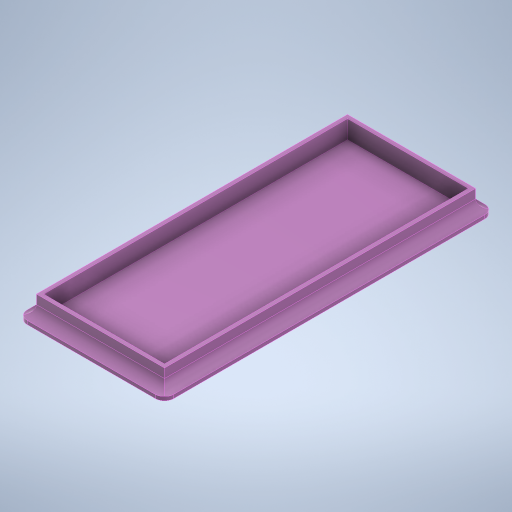
# Autodesk Inventor part: hodnky3-horní
Saved by Autodesk Inventor 2023.2 (Build 272271000, 271)
## iProperties
Created: 2024-01-21
Part Number: hodnky3-horní
Material: Generic
Document SubType Name: Modeling
Designer: marek
Density: 1 g/cm^3
Appearance: Smooth - Purple
Author: marek
Autodesk Inventor part; units mm, degrees
ref_plane "YZ Plane" through (0, 0, 0) normal (1, 0, 0) x (0, 1, 0)
ref_plane "XZ Plane" through (0, 0, 0) normal (0, 1, 0) x (-1, 0, 0)
ref_plane "XY Plane" through (0, 0, 0) normal (0, 0, 1) x (1, 0, 0)
sketch "Sketch1" plane through (0, 0, 0) normal (0, 1, 0) x (-1, 0, 0)
  line L0 (20, -45) -> (-20, -45)
  line L1 (-20, -45) -> (-20, 45)
  line L2 (-20, 45) -> (20, 45)
  line L3 (20, 45) -> (20, -45)
  line L4 (0, -63) -> (0, 63) projected
  line L5 (-28, 0) -> (28, 0) projected
  point P0 (0, 0)
  dimension "d0" = 40
  dimension "d1" = 90
  constraints: 8 end point, 2 parallel, 1 horizontal, 1 perpendicular, 2 other
  measures "d0" distance of L2.end L1.end
  measures "d1" distance of L1.end L0.end
extrude "Extrusion1" add sketch "Sketch1" along normal blind 1
sketch "Sketch2" plane through (0, 1, 0) normal (0, 1, 0) x (1, 0, 0)
  line L0 (20, -45) -> (20, 45) projected
  line L1 (-20, -45) -> (20, -45) projected
  line L2 (-20, 45) -> (-20, -45) projected
  line L3 (20, 45) -> (-20, 45) projected
  line L4 (-16.5, -41.5) -> (16.5, -41.5)
  line L5 (16.5, -41.5) -> (16.5, 41.5)
  line L6 (16.5, 41.5) -> (-16.5, 41.5)
  line L7 (-16.5, 41.5) -> (-16.5, -41.5)
  line L8 (-17.5, -42.5) -> (17.5, -42.5)
  line L9 (17.5, -42.5) -> (17.5, 42.5)
  line L10 (17.5, 42.5) -> (-17.5, 42.5)
  line L11 (-17.5, 42.5) -> (-17.5, -42.5)
  point P0 (0, 0)
  dimension "d4" = 3.5
  dimension "d5" = 1
  constraints: 16 end point, 6 other
  measures "d4" distance between parallel lines of L2 L7
  measures "d5" distance between parallel lines of L7 L11
extrude "Extrusion2" add sketch "Sketch2" along normal blind 5 contours L11 L10 L9 L8
fillet "Face Fillet1" radius 2.5 1 edges at (0, 1, 42.5)
fillet "Face Fillet2" radius 2.5 1 edges at (17.5, 1, 0)
fillet "Face Fillet3" radius 2.5 1 edges at (-17.5, 1, 0)
fillet "Face Fillet4" radius 2.5 1 edges at (0, 1, -42.5)
fillet "Fillet1" radius 2.5 4 edges at (-20, 0.5, -45) (-20, 0.5, 45) (20, 0.5, -45) (20, 0.5, 45)
sketch "Sketch3" plane through (0, 0, 0) normal (0, -1, 0) x (1, 0, 0)
  line L0 (-1.5, -37.7) -> (1.5, -37.7)
  line L1 (1.5, -37.7) -> (1.5, -26.7)
  line L2 (1.5, -26.7) -> (-1.5, -26.7)
  line L3 (-1.5, -26.7) -> (-1.5, -37.7)
  line L4 (0, 63.0032) -> (0, -63.0032) projected
  line L5 (-28.0032, 0) -> (28.0032, 0) projected
  line L6 (17.5, -45) -> (-17.5, -45) projected
  line L7 (-1.5, -5.5) -> (1.5, -5.5)
  line L8 (1.5, -5.5) -> (1.5, 5.5)
  line L9 (1.5, 5.5) -> (-1.5, 5.5)
  line L10 (-1.5, 5.5) -> (-1.5, -5.5)
  line L11 (-1.5, 26.7) -> (1.5, 26.7)
  line L12 (1.5, 26.7) -> (1.5, 37.7)
  line L13 (1.5, 37.7) -> (-1.5, 37.7)
  line L14 (-1.5, 37.7) -> (-1.5, 26.7)
  line L15 (-17.5, 45) -> (17.5, 45) projected
  point P0 (0, 0)
  dimension "d13" = 11
  dimension "d14" = 3
  dimension "d15" = 7.3
  dimension "d16" = 11
  dimension "d17" = 3
  dimension "d18" = 11
  dimension "d19" = 3
  dimension "d20" = 21.2
  dimension "d21" = 21.2
  dimension "d22" = 7.3
  constraints: 24 end point, 9 parallel, 3 horizontal, 3 perpendicular, 1 other
  measures "d13" distance of L1.end L0.end
  measures "d14" distance of L1.end L2.end
  measures "d15" distance between parallel lines of L6 L0
  measures "d16" distance of L8.end L7.end
  measures "d17" distance of L8.end L9.end
  measures "d18" distance of L12.end L11.end
  measures "d19" distance of L12.end L13.end
  measures "d20" distance between parallel lines of L2 L7
  measures "d21" distance between parallel lines of L11 L9
  measures "d22" distance between parallel lines of L15 L13
extrude "Extrusion3" add sketch "Sketch3" along normal blind 1
sketch "Sketch4" plane through (1.5, 0, 5.5) normal (1, 0, 0) x (0, 0, -1)
  line L0 (-37, 0) -> (48, 0) projected
  line L1 (-31.7, 0) -> (-21.7, 0)
  line L2 (-21.7, 0) -> (-21.7, -0.5)
  line L3 (-21.7, -0.5) -> (-31.7, -0.5)
  line L4 (-31.7, -0.5) -> (-31.7, 0)
  line L5 (0, 0) -> (11, 0) projected
  line L6 (0.5, 0) -> (10.5, 0)
  line L7 (10.5, 0) -> (10.5, -0.5)
  line L8 (10.5, -0.5) -> (0.5, -0.5)
  line L9 (0.5, -0.5) -> (0.5, 0)
  line L10 (32.7, 0) -> (42.7, 0)
  line L11 (42.7, 0) -> (42.7, -0.5)
  line L12 (42.7, -0.5) -> (32.7, -0.5)
  line L13 (32.7, -0.5) -> (32.7, 0)
  line L14 (-32.2, 0) -> (-32.2, -1) projected
  line L15 (-21.2, -1) -> (-32.2, -1) projected
  line L16 (-21.2, 0) -> (-21.2, -1) projected
  line L17 (0, 0) -> (0, -1) projected
  line L18 (11, -1) -> (0, -1) projected
  line L19 (11, 0) -> (11, -1) projected
  line L20 (32.2, 0) -> (32.2, -1) projected
  line L21 (43.2, -1) -> (32.2, -1) projected
  line L22 (43.2, 0) -> (43.2, -1) projected
  point P0 (5.5, 0)
  point P1 (0, -0.5)
  point P2 (0.5, 0)
  dimension "d25" = 0.5
  dimension "d26" = 0.5
  dimension "d27" = 0.5
  dimension "d29" = 0.5
  dimension "d30" = 0.5
  dimension "d31" = 0.5
  dimension "d32" = 0.5
  dimension "d33" = 0.5
  dimension "d34" = 0.5
  constraints: 24 end point, 6 parallel, 3 horizontal, 3 perpendicular, 1 midpoint, 1 point on line, 3 other
  measures "d25" distance between parallel lines of L14 L4
  measures "d26" distance between parallel lines of L15 L3
  measures "d27" distance between parallel lines of L16 L2
  measures "d29" distance between parallel lines of L9 L17
  measures "d30" distance between parallel lines of L8 L18
  measures "d31" distance between parallel lines of L19 L7
  measures "d32" distance between parallel lines of L20 L13
  measures "d33" distance between parallel lines of L21 L12
  measures "d34" distance between parallel lines of L22 L11
extrude "Extrusion4" cut sketch "Sketch4" against normal up to surface (3 mm away) contours L0 L2 L3 L4 | L0 L7 L8 L9 | L0 L11 L12 L13
fillet "Fillet2" radius 0.5 6 edges at (0, -1, 37.7) (0, -1, 26.7) (0, -1, 5.5) (0, -1, -5.5) (0, -1, -26.7) (0, -1, -37.7)
body "Solid1"
